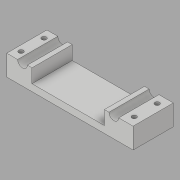
# Autodesk Inventor part: g_servo mount 2
Saved by Autodesk Inventor 2019 (Build 230136000, 136)
## iProperties
Created: 2021-10-30
Part Number: g_servo mount 2
Material: Generic
Document SubType Name: Modeling
Designer: Mohamed
Density: 1 g/cm^3
Appearance: Default
Author: Mohamed
Autodesk Inventor part; units mm, degrees
ref_plane "YZ Plane" through (0, 0, 0) normal (1, 0, 0) x (0, 1, 0)
ref_plane "XZ Plane" through (0, 0, 0) normal (0, 1, 0) x (-1, 0, 0)
ref_plane "XY Plane" through (0, 0, 0) normal (0, 0, 1) x (1, 0, 0)
sketch "Sketch1" plane through (0, 0, 0) normal (0, 0, 1) x (1, 0, 0)
  line L0 (0, 0) -> (110, 0)
  line L1 (110, 0) -> (110, 18)
  line L2 (110, 18) -> (97.5, 18)
  arc A0 (89, 18) -> (97.5, 18) centre (93.25, 18) ccw
  line L3 (89, 18) -> (85, 18)
  line L4 (85, 18) -> (85, 6)
  line L5 (85, 6) -> (22, 6)
  line L6 (22, 6) -> (22, 18)
  line L7 (22, 18) -> (18, 18)
  arc A1 (9.5, 18) -> (18, 18) centre (13.75, 18) ccw
  line L8 (9.5, 18) -> (0, 18)
  line L9 (0, 18) -> (0, 0)
  dimension "d0" = 110
  dimension "d1" = 18
  dimension "d2" = 12.5
  dimension "d4" = 8.5
  dimension "d5" = 4
  dimension "d6" = 12
  dimension "d7" = 63
  dimension "d8" = 12
  dimension "d9" = 4
  dimension "d11" = 8.5
  constraints: 20 end point, 5 horizontal, 4 perpendicular, 4 point on circle, 2 centre point, 1 vertical
  measures "d0" distance of L0.start L0.end
  measures "d1" distance of L0.end L1.end
  measures "d2" distance of L1.end L2.end
  measures "d4" diameter of A0
  measures "d5" distance of L3.start L3.end
  measures "d6" distance of L3.end L4.end
  measures "d7" distance of L4.end L5.end
  measures "d8" distance of L5.end L6.end
  measures "d9" distance of L6.end L7.end
  measures "d11" diameter of A1
extrude "Extrusion1" add sketch "Sketch1" against normal blind 35
sketch "Sketch2" plane through (97.5, 18, 0) normal (0, 1, 0) x (1, 0, 0)
  line L0 (12.5, 0) -> (12.5, 35) projected
  circle A0 centre (6, 27.5) radius 2
  circle A1 centre (6, 7.5) radius 2
  line L1 (-97.5, 0) -> (-97.5, 35) projected
  circle A2 centre (-92.5, 27.5) radius 2
  circle A3 centre (-92.5, 7.5) radius 2
  dimension "d17" = 4
  dimension "d18" = 4
  dimension "d22" = 4
  dimension "d23" = 4
  constraints: 4 centre point
  measures "d17" diameter of A0
  measures "d18" diameter of A1
  measures "d22" diameter of A2
  measures "d23" diameter of A3
extrude "Extrusion2" cut sketch "Sketch2" against normal blind 18
body "Solid1"
